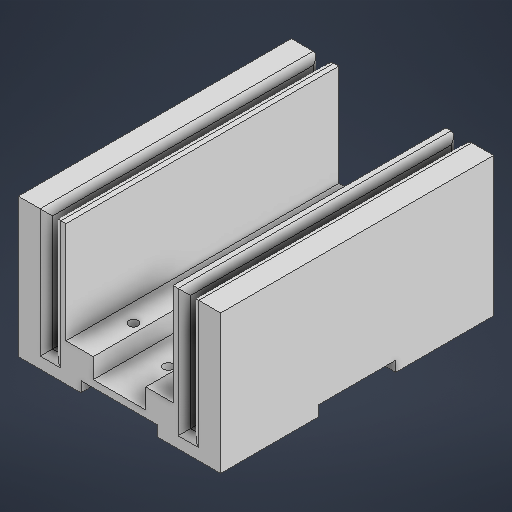
# Autodesk Inventor part: slider
Saved by Autodesk Inventor 2026.2 (Build 302298000, 298)
## iProperties
Created: 2026-04-06
Part Number: slider
Material: Generic
Document SubType Name: Modeling
Designer: Brian Wang
Density: 1 g/cm^3
Appearance: Default
Author: Brian Wang
Autodesk Inventor part; units mm, degrees
ref_plane "YZ Plane" through (0, 0, 0) normal (1, 0, 0) x (0, 1, 0)
ref_plane "XZ Plane" through (0, 0, 0) normal (0, 1, 0) x (-1, 0, 0)
ref_plane "XY Plane" through (0, 0, 0) normal (0, 0, 1) x (1, 0, 0)
sketch "Sketch1" plane through (0, 0, 0) normal (0, 1, 0) x (-1, 0, 0)
  line L0 (9.1683, 14.0813) -> (-48.6317, 14.0813)
  line L1 (-48.6317, 14.0813) -> (-48.6317, -63.9187)
  line L2 (-48.6317, -63.9187) -> (9.1683, -63.9187)
  line L3 (9.1683, -63.9187) -> (9.1683, 14.0813)
  point P0 (0, 0)
  dimension "d0" = 57.8
  dimension "d1" = 78
  constraints: 8 end point, 2 parallel, 1 horizontal, 1 perpendicular
  measures "d0" distance of L2.end L1.end
  measures "d1" distance of L1.end L0.end
extrude "Extrusion1" add sketch "Sketch1" along normal blind 2
sketch "Sketch2" plane through (0, 2, 0) normal (0, 1, 0) x (1, 0, 0)
  line L0 (-9.1683, 63.9187) -> (-9.1683, -14.0813) projected
  line L1 (48.6317, 63.9187) -> (-9.1683, 63.9187) projected
  line L2 (-9.1683, -14.0813) -> (-1.1683, -14.0813)
  line L3 (-1.1683, -14.0813) -> (-1.1683, 63.9187)
  line L4 (-1.1683, 63.9187) -> (-9.1683, 63.9187)
  line L5 (-9.1683, 63.9187) -> (-9.1683, -14.0813)
  line L6 (48.6317, -14.0813) -> (48.6317, 63.9187) projected
  line L7 (48.6317, -14.0813) -> (40.6317, -14.0813)
  line L8 (40.6317, -14.0813) -> (40.6317, 63.9187)
  line L9 (40.6317, 63.9187) -> (48.6317, 63.9187)
  line L10 (48.6317, 63.9187) -> (48.6317, -14.0813)
  line L11 (1.2317, -14.0813) -> (1.2317, 63.9187)
  line L12 (-9.1683, -14.0813) -> (48.6317, -14.0813) projected
  line L13 (38.2317, -14.0813) -> (38.2317, 63.9187)
  line L14 (1.2317, -14.0813) -> (38.2317, -14.0813)
  line L15 (1.2317, 63.9187) -> (38.2317, 63.9187)
  point P0 (0, 0)
  dimension "d4" = 8
  dimension "d5" = 8
  dimension "d6" = 2.4
  dimension "d7" = 2.4
  constraints: 24 end point, 5 perpendicular, 5 point on line, 4 parallel, 2 horizontal, 1 collinear
  measures "d4" distance of L4.end L3.end
  measures "d5" distance of L8.end L9.end
  measures "d6" distance between parallel lines of L3 L11
  measures "d7" distance between parallel lines of L8 L13
extrude "Extrusion2" add sketch "Sketch2" along normal blind 5.7 contours L1 L3 L2 L0 | L1 L13 L12 L11 | L1 L6 L7 L8
sketch "Sketch3" plane through (0, 7.7, 0) normal (0, 1, 0) x (1, 0, 0)
  circle A0 centre (9.7317, -0.0813) radius 1.35
  circle A1 centre (29.7317, -0.0813) radius 1.35
  line L0 (1.2317, 63.9187) -> (1.2317, -14.0813) projected
  circle A2 centre (9.7317, 49.9187) radius 1.35
  circle A3 centre (29.7317, 49.9187) radius 1.35
  line L1 (1.2317, -14.0813) -> (38.2317, -14.0813) projected
  point P0 (0, 0)
  dimension "d10" = 2.7
  dimension "d11" = 2.7
  dimension "d12" = 20
  dimension "d13" = 8.5
  dimension "d14" = 2.7
  dimension "d15" = 2.7
  dimension "d16" = 20
  dimension "d17" = 50
  dimension "d18" = 14
  dimension "d19" = 14
  dimension "d20" = 50
  constraints: 4 centre point
  measures "d10" diameter of A0
  measures "d11" diameter of A1
  measures "d12" distance of A1.centre A0.centre
  measures "d13" distance from line of L0 A0.centre
  measures "d14" diameter of A2
  measures "d15" diameter of A3
  measures "d16" distance of A3.centre A2.centre
  measures "d17" distance of A0.centre A2.centre
  measures "d18" distance from line of L1 A0.centre
  measures "d19" distance from line of L1 A1.centre
  measures "d20" distance of A1.centre A3.centre
extrude "Extrusion3" cut sketch "Sketch3" against normal through all
sketch "Sketch4" plane through (0, 0, 0) normal (0, -1, 0) x (1, 0, 0)
  line L0 (8.7317, 14.0813) -> (8.7317, -13.9187)
  line L1 (8.7317, -13.9187) -> (-9.1683, -13.9187)
  line L2 (-9.1683, -35.9187) -> (8.7317, -35.9187)
  line L3 (8.7317, -35.9187) -> (8.7317, -63.9187)
  line L4 (8.7317, -63.9187) -> (30.7317, -63.9187)
  line L5 (30.7317, -63.9187) -> (30.7317, -35.9187)
  line L6 (30.7317, -35.9187) -> (48.6317, -35.9187)
  line L7 (48.6317, -13.9187) -> (30.7317, -13.9187)
  line L8 (30.7317, 14.0813) -> (30.7317, -13.9187)
  line L9 (30.7317, 14.0813) -> (8.7317, 14.0813)
  circle A0 centre (19.7317, 0.0813) radius 1.375
  circle A1 centre (19.7317, -49.9187) radius 1.375
  line L10 (48.6317, 14.0813) -> (48.6317, -63.9187) projected
  line L11 (-9.1683, 14.0813) -> (48.6317, 14.0813) projected
  line L12 (-9.1683, -13.9187) -> (-9.1683, -35.9187)
  line L13 (-9.1683, -63.9187) -> (-9.1683, 14.0813) projected
  line L14 (48.6317, -13.9187) -> (48.6317, -35.9187)
  line L15 (-9.1683, 14.0813) -> (48.6317, 14.0813)
  line L16 (48.6317, 14.0813) -> (48.6317, -63.9187)
  line L17 (48.6317, -63.9187) -> (-9.1683, -63.9187)
  line L18 (-9.1683, -63.9187) -> (-9.1683, 14.0813)
  point P0 (0, 0)
  point P1 (24.2887, -20.9845)
  point P2 (19.7317, -63.9187)
  dimension "d48" = 17.9
  dimension "d49" = 17.9
  dimension "d50" = 28
  dimension "d52" = 28
  dimension "d53" = 22
  dimension "d70" = 0
  constraints: 32 end point, 10 point on line, 6 perpendicular, 2 centre point, 2 parallel, 1 horizontal, 1 midpoint, 1 vertical alignment
  measures "d48" distance between parallel lines of L13 L0
  measures "d49" distance between parallel lines of L16 L8
  measures "d50" distance between parallel lines of L11 L1
  measures "d52" distance between parallel lines of L17 L2
  measures "d53" distance of L7.start L6.end
  measures "d70" horizontal distance of point (19.732, -63.919) A1.centre
extrude "Extrusion4" add sketch "Sketch4" along normal blind 3 contours L0 L1 L13 L11 | L11 L10 L7 L8 | L2 L3 L17 L13 | L10 L17 L5 L6 | A0 | A1
sketch "Sketch5" plane through (24.7317, -3, 0.0813) normal (0, -1, 0) x (1, 0, 0)
  circle A0 centre (-5, 0) radius 1.375 projected
  circle A1 centre (-5, 0) radius 1.375
  circle A2 centre (-5, -50) radius 1.375 projected
  circle A3 centre (-5, -50) radius 1.375
  point P0 (-24.7317, -0.0813)
  dimension "d56" = 2.75
  constraints: 2 centre point, 2 coincident
  measures "d56" diameter of A1
extrude "Extrusion5" cut sketch "Sketch5" against normal through all
sketch "Sketch6" plane through (0, 7.7, 0) normal (0, 1, 0) x (1, 0, 0)
  line L0 (12.2317, 63.9187) -> (27.2317, 63.9187)
  line L1 (27.2317, 63.9187) -> (27.2317, -14.0813)
  line L2 (27.2317, -14.0813) -> (12.2317, -14.0813)
  line L3 (12.2317, -14.0813) -> (12.2317, 63.9187)
  line L4 (38.2317, 63.9187) -> (1.2317, 63.9187) projected
  line L5 (1.2317, -14.0813) -> (38.2317, -14.0813) projected
  line L6 (48.6317, -14.0813) -> (48.6317, 63.9187) projected
  line L7 (-9.1683, 63.9187) -> (-9.1683, -14.0813) projected
  point P0 (0, 0)
  dimension "d59" = 0
  dimension "d60" = 0
  dimension "d61" = 21.4
  dimension "d62" = 21.4
  constraints: 8 end point, 2 parallel, 1 horizontal, 1 perpendicular
  measures "d59" distance between parallel lines of L4 L0
  measures "d60" distance between parallel lines of L5 L2
  measures "d61" distance between parallel lines of L6 L1
  measures "d62" distance between parallel lines of L7 L3
extrude "Extrusion6" cut sketch "Sketch6" against normal blind 5.7
sketch "Sketch7" plane through (0, 7.7, 0) normal (0, 1, 0) x (1, 0, 0)
  line L0 (-9.1683, 63.9187) -> (-9.1683, -14.0813) projected
  line L1 (-1.1683, -14.0813) -> (1.2317, -14.0813) projected
  line L2 (-9.1683, 63.9187) -> (-1.1683, 63.9187)
  line L3 (-1.1683, 63.9187) -> (-1.1683, -14.0813)
  line L4 (-1.1683, -14.0813) -> (-9.1683, -14.0813)
  line L5 (-9.1683, -14.0813) -> (-9.1683, 63.9187)
  line L6 (48.6317, -14.0813) -> (48.6317, 63.9187) projected
  line L7 (40.6317, -14.0813) -> (40.6317, 63.9187) projected
  line L8 (48.6317, -14.0813) -> (40.6317, -14.0813)
  line L9 (40.6317, -14.0813) -> (40.6317, 63.9187)
  line L10 (40.6317, 63.9187) -> (48.6317, 63.9187)
  line L11 (48.6317, 63.9187) -> (48.6317, -14.0813)
  line L12 (1.2317, -14.0813) -> (1.2317, 63.9187) projected
  line L13 (1.2317, 63.9187) -> (4.4317, 63.9187)
  line L14 (4.4317, 63.9187) -> (4.4317, -14.0813)
  line L15 (4.4317, -14.0813) -> (1.2317, -14.0813)
  line L16 (1.2317, -14.0813) -> (1.2317, 63.9187)
  line L17 (38.2317, 63.9187) -> (38.2317, -14.0813) projected
  line L18 (38.2317, 63.9187) -> (35.0317, 63.9187)
  line L19 (35.0317, 63.9187) -> (35.0317, -14.0813)
  line L20 (35.0317, -14.0813) -> (38.2317, -14.0813)
  line L21 (38.2317, -14.0813) -> (38.2317, 63.9187)
  point P0 (0, 0)
  point P1 (38.2317, -14.0813)
  dimension "d71" = 3.2
  dimension "d72" = 3.2
  constraints: 32 end point, 8 parallel, 4 horizontal, 4 perpendicular, 2 point on line
  measures "d71" distance of L14.end L15.end
  measures "d72" distance of L20.end L19.end
extrude "Extrusion7" add sketch "Sketch7" along normal blind 29
fillet "Fillet6" radius 1.765 16 edges at (-1.1683, 19.35, 14.0813) (1.2317, 19.35, 14.0813) (1.2317, 36.7, -24.9187) (-1.1683, 36.7, -24.9187) (0.0317, 2, 14.0813) (38.2317, 36.7, -24.9187) (40.6317, 36.7, -24.9187) (38.2317, 19.35, 14.0813) (40.6317, 19.35, 14.0813) (39.4317, 2, 14.0813) (-1.1683, 19.35, -63.9187) (1.2317, 19.35, -63.9187) (38.2317, 19.35, -63.9187) (40.6317, 19.35, -63.9187) (39.4317, 2, -63.9187) (0.0317, 2, -63.9187)
body "Solid1"
